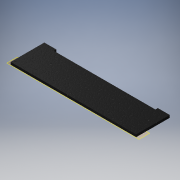
# Autodesk Inventor part: sides
Saved by Autodesk Inventor 2018 (Build 220112000, 112)
## iProperties
Created: 2017-10-09
Part Number: sides
Material: Generic
Document SubType Name: Modeling
Designer: HP
Density: 1 g/cm^3
Appearance: Fine Textured - Black
Author: HP
Autodesk Inventor part; units mm, degrees
ref_plane "YZ Plane" through (0, 0, 0) normal (1, 0, 0) x (0, 1, 0)
ref_plane "XZ Plane" through (0, 0, 0) normal (0, 1, 0) x (-1, 0, 0)
ref_plane "XY Plane" through (0, 0, 0) normal (0, 0, 1) x (1, 0, 0)
ref_plane "Work Plane1" through (0, 0, 0.5) normal (0, 0, 1) x (1, 0, 0)
sketch "Sketch1" plane through (0, 0, 0.5) normal (0, 0, 1) x (1, 0, 0)
  line L0 (250, 0) -> (0, 0) construction
  line L1 (250, 0) -> (250, 20) construction
  line L2 (0, 20) -> (250, 20) construction
  line L3 (0, 0) -> (0, 20) construction
  line L4 (245, 20) -> (153.1686, 20) construction
  line L5 (245, 20) -> (245, 80) construction
  line L6 (153.1686, 80) -> (245, 80) construction
  line L7 (153.1686, 20) -> (153.1686, 80) construction
  line L8 (-5.5, 0) -> (255.5, 0)
  line L9 (255.5, 0) -> (255.5, 70)
  line L10 (255.5, 70) -> (230.6, 70)
  line L11 (230.6, 70) -> (230.6, 64.9)
  line L12 (230.6, 64.9) -> (19.4, 64.9)
  line L13 (19.4, 64.9) -> (19.4, 70)
  line L14 (19.4, 70) -> (-5.5, 70)
  line L15 (-5.5, 70) -> (-5.5, 0)
  dimension "d0" = 10
  dimension "d1" = 5.1
  dimension "d2" = 5.5
  dimension "d3" = 5.5
  dimension "d4" = 24.9
  dimension "d5" = 24.9
  constraints: 18 end point, 5 perpendicular, 3 point on line, 1 collinear, 1 vertical
  measures "d0" distance between parallel lines of L10 L6
  measures "d1" distance between parallel lines of L12 L10
  measures "d2" distance between parallel lines of L15 L3
  measures "d3" distance between parallel lines of L9 L1
  measures "d4" distance between parallel lines of L13 L15
  measures "d5" distance between parallel lines of L11 L9
extrude "Extrusion1" add sketch "Sketch1" along normal blind 5
hole "Hole1" [suppressed]
hole "Hole2" [suppressed]
sketch "Sketch2" plane through (0, 0, 0.5) normal (0, 0, -1) x (-1, 0, 0)
  line L0 (0, 0) -> (-250, 0) construction
  line L1 (0, 0) -> (0, 20) construction
  line L2 (-250, 20) -> (0, 20) construction
  line L3 (-250, 0) -> (-250, 20) construction
  line L4 (5.5, 0) -> (-255.5, 0) construction
  line L5 (5.5, 70) -> (5.5, 0) construction
  line L6 (-19.4, 70) -> (5.5, 70) construction
  line L7 (-19.4, 64.9) -> (-19.4, 70) construction
  line L8 (-230.6, 64.9) -> (-19.4, 64.9) construction
  line L9 (-230.6, 70) -> (-230.6, 64.9) construction
  line L10 (-255.5, 70) -> (-230.6, 70) construction
  line L11 (-255.5, 0) -> (-255.5, 70) construction
  line L12 (-125, 20) -> (-125, 0) construction
  line L13 (-250, 10) -> (0, 10) construction
  point P0 (-125, 10)
  point P1 (-230, 10)
  point P2 (-20, 10)
  dimension "d30" = 20
  dimension "d31" = 20
  constraints: 5 midpoint, 4 end point, 2 point on line
  measures "d30" distance from line of point (-230, 10) L3
  measures "d31" distance from line of point (-20, 10) L1
hole "Hole3" at (125, 10, 0.5) at (230, 10, 0.5) at (20, 10, 0.5) direction (0, 0, 1) diameter 5 end through all
equation "\"d1\" = ABS_tolerance + plate_thickness"
equation "\"d2\" = plate_thickness + basic_plate_offset"
equation "\"d3\" = plate_thickness + basic_plate_offset"
equation "\"d5\" = d4"
equation "\"d6\" = plate_thickness"
equation "\"plate_thickness\" = 5"
equation "\"ABS_tolerance\" = 0.1"
equation "\"laser_cutter_thickness\" = 0.1"
equation "\"basic_plate_offser\" = 0.5"
equation "\"basic_plate_offset\" = 0.5"
body "Solid1"
